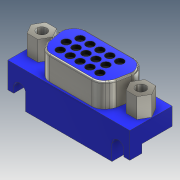
# Autodesk Inventor part: db15-connector-pcb
Saved by Autodesk Inventor 2017 (Build 210142000, 142)
## iProperties
Created: 2018-07-16
Part Number: db15-connector-pcb
Material: Generic
Document SubType Name: Modeling
Designer: Luiz Gustavo
Density: 1 g/cm^3
Appearance: Default
Author: Luiz Gustavo
Autodesk Inventor part; units mm, degrees
ref_plane "YZ Plane" through (0, 0, 0) normal (1, 0, 0) x (0, 1, 0)
ref_plane "XZ Plane" through (0, 0, 0) normal (0, 1, 0) x (-1, 0, 0)
ref_plane "XY Plane" through (0, 0, 0) normal (0, 0, 1) x (1, 0, 0)
sketch "Sketch1" plane through (0, 0, 0) normal (0, 0, 1) x (1, 0, 0)
  line L0 (-15.4, 5.35) -> (15.4, 5.35)
  line L1 (15.4, 5.35) -> (15.4, -5.35)
  line L2 (15.4, -5.35) -> (-15.4, -5.35)
  line L3 (-15.4, -5.35) -> (-15.4, 5.35)
  line L4 (-15.4, 5.35) -> (15.4, -5.35) construction
  line L5 (15.4, 5.35) -> (-15.4, -5.35) construction
  line L6 (-15.4, 0.35) -> (15.4, 0.35) construction
  circle A0 centre (-12.5, 0.35) radius 1.25
  circle A1 centre (12.5, 0.35) radius 1.25
  line L7 (0, 5.35) -> (0, -5.35) construction
  circle A2 centre (-12.5, 0.35) radius 2.7424 construction
  line L8 (-13.8712, -2.025) -> (-11.1288, 2.725) construction
  line L9 (-13.8712, 2.725) -> (-11.1288, -2.025) construction
  line L10 (-9.7576, 0.35) -> (-15.2424, 0.35) construction
  line L11 (-11.1288, 2.725) -> (-13.8712, 2.725)
  line L12 (-13.8712, 2.725) -> (-15.2424, 0.35)
  line L13 (-15.2424, 0.35) -> (-13.8712, -2.025)
  line L14 (-13.8712, -2.025) -> (-11.1288, -2.025)
  line L15 (-11.1288, -2.025) -> (-9.7576, 0.35)
  line L16 (-9.7576, 0.35) -> (-11.1288, 2.725)
  line L17 (11.1288, 2.725) -> (13.8712, 2.725)
  line L18 (13.8712, 2.725) -> (15.2424, 0.35)
  line L19 (15.2424, 0.35) -> (13.8712, -2.025)
  line L20 (13.8712, -2.025) -> (11.1288, -2.025)
  line L21 (11.1288, -2.025) -> (9.7576, 0.35)
  line L22 (9.7576, 0.35) -> (11.1288, 2.725)
  line L23 (-7.5, 5.15) -> (7.5, 5.15)
  line L24 (7.5, 5.15) -> (9.5, 2.55)
  line L25 (9.5, 2.55) -> (8.5, -2.65)
  line L26 (8.5, -2.65) -> (6.75, -4.85)
  line L27 (6.75, -4.85) -> (-6.75, -4.85)
  line L28 (-6.75, -4.85) -> (-8.5, -2.65)
  line L29 (-8.5, -2.65) -> (-9.5, 2.55)
  line L30 (-9.5, 2.55) -> (-7.5, 5.15)
  point P0 (0, 0)
  dimension "d0" = 30.8
  dimension "d1" = 10.7
  dimension "d2" = 2.5
  dimension "d4" = 60
  dimension "d5" = 60
  dimension "d6" = 4.75
  dimension "d7" = 5
  dimension "d8" = 25
  dimension "d9" = 15
  dimension "d10" = 19
  dimension "d11" = 13.5
  dimension "d12" = 17
  dimension "d13" = 10
  dimension "d14" = 7.4
  dimension "d15" = 2.2
  dimension "d16" = 0.2
  constraints: 62 end point, 10 symmetric about line, 7 midpoint, 6 parallel, 6 point on circle, 4 horizontal, 4 point on line, 3 centre point, 1 perpendicular, 1 other
  measures "d0" distance of L1.end L2.end
  measures "d1" distance of L0.end L1.end
  measures "d2" diameter of A0
  measures "d4" angle of L9 L8
  measures "d5" angle of L9 L10
  measures "d6" distance between parallel lines of L14 L11
  measures "d7" distance between parallel lines of L6 L0
  measures "d8" distance of A1.centre A0.centre
  measures "d9" distance of L23.start L23.end
  measures "d10" distance of L24.end L29.end
  measures "d11" distance of L26.end L27.end
  measures "d12" distance of L25.end L28.end
  measures "d13" distance between parallel lines of L27 L23
  measures "d14" distance from line of L29.end L27
  measures "d15" vertical distance of L26.end L25.end
  measures "d16" distance between parallel lines of L23 L0
extrude "Extrusion1" add sketch "Sketch1" along normal blind 5 contours L16 L15 L14 L13 L12 L11 | L17 L18 L19 L20 L21 L22
extrude "Extrusion2" add sketch "Sketch1" along normal blind 6 contours L23 L24 L25 L26 L27 L28 L29 L30
extrude "Extrusion3" add sketch "Sketch1" against normal blind 9 contours L0 L1 L2 L3 | A0 | A1 | L16 L15 L14 L13 L12 L11 | L17 L18 L19 L20 L21 L22 | L23 L24 L25 L26 L27 L28 L29 L30
sketch "Sketch2" plane through (-15.4, 5.35, 0) normal (0, 1, 0) x (1, 0, 0)
  line L0 (0, 0) -> (30.8, 0) projected
  line L1 (30.8, 0) -> (30.8, 9) projected
  line L2 (0, 9) -> (30.8, 9) projected
  line L3 (0, 0) -> (0, 9) projected
  line L4 (15.4, 0) -> (15.4, 9) construction
  line L5 (0, 0) -> (0, 9) projected
  line L6 (0, 9) -> (6.9, 9)
  line L7 (6.9, 9) -> (6.9, 4.4)
  line L8 (6.9, 4.4) -> (0, 4.4)
  line L9 (0, 4.4) -> (0, 9)
  line L10 (30.8, 9) -> (0, 9) projected
  line L11 (30.8, 9) -> (23.9, 9)
  line L12 (23.9, 9) -> (23.9, 4.4)
  line L13 (23.9, 4.4) -> (30.8, 4.4)
  line L14 (30.8, 4.4) -> (30.8, 9)
  line L15 (6.9, 4.4) -> (23.9, 4.4) construction
  dimension "d23" = 17
  dimension "d24" = 4.4
  constraints: 20 end point, 4 parallel, 3 perpendicular, 2 horizontal, 1 midpoint, 1 point on line, 1 other
  measures "d23" distance between parallel lines of L12 L7
  measures "d24" distance between parallel lines of L0 L15
extrude "Extrusion4" cut sketch "Sketch2" against normal blind 7.7 contours L3 L2 L7 L8 | L13 L12 L2 L1
sketch "Sketch3" plane through (0, 0, 6) normal (0, 0, 1) x (1, 0, 0)
  line L0 (-5, 2.5) -> (3.2977, 2.5) construction
  circle A0 centre (-5, 2.5) radius 1
  circle A1 centre (-2.5, 2.5) radius 1
  circle A2 centre (0, 2.5) radius 1
  circle A3 centre (2.5, 2.5) radius 1
  circle A4 centre (5, 2.5) radius 1
  line L1 (-6, 0) -> (3.7977, 0) construction
  circle A5 centre (-6, 0) radius 1
  circle A6 centre (-3.5, 0) radius 1
  circle A7 centre (-1, 0) radius 1
  circle A8 centre (1.5, 0) radius 1
  circle A9 centre (4, 0) radius 1
  line L2 (-5, -2.5) -> (3.1289, -2.5) construction
  circle A10 centre (-5, -2.5) radius 1
  circle A11 centre (-2.5, -2.5) radius 1
  circle A12 centre (0, -2.5) radius 1
  circle A13 centre (2.5, -2.5) radius 1
  circle A14 centre (5, -2.5) radius 1
  line L3 (0, 2.5) -> (0, -2.5) construction
  point P0 (0, 0)
  point P1 (0, 0)
  dimension "d27" = 2
  dimension "d30" = 2.5
  dimension "d39" = 2
  dimension "d40" = 2.5
  dimension "d50" = 2
  dimension "d51" = 2.5
  dimension "d53" = 2.5
  dimension "d54" = 2.5
  constraints: 15 centre point, 8 end point, 6 horizontal, 4 coincident, 1 midpoint, 1 tangent, 1 vertical, 24 other
  measures "d27" diameter of A0
  measures "d30" distance of A0.centre A1.centre
  measures "d39" diameter of A5
  measures "d40" distance of A5.centre A6.centre
  measures "d50" diameter of A10
  measures "d51" distance of A10.centre A11.centre
  measures "d53" vertical distance of A9.centre A4.centre
  measures "d54" vertical distance of A14.centre A9.centre
extrude "Extrusion5" cut sketch "Sketch3" against normal blind 1
fillet "Fillet1" radius 3 8 edges at (-7.5, 5.15, 3) (-9.5, 2.55, 3) (-8.5, -2.65, 3) (-6.75, -4.85, 3) (6.75, -4.85, 3) (8.5, -2.65, 3) (9.5, 2.55, 3) (7.5, 5.15, 3)
sketch "Sketch4" plane through (0, 0, 0) normal (0, 1, 0) x (-1, 0, 0)
  line L0 (-15.4, -9) -> (15.4, -9) projected
  line L1 (15.4, -4.4) -> (15.4, -9) projected
  line L2 (-15.4, -9) -> (-15.4, -4.4) projected
  line L3 (15.4, -6.5) -> (13.9, -6.5)
  line L4 (13.9, -6.5) -> (13.9, -5)
  line L5 (10.9, -5) -> (10.9, -9)
  line L6 (10.9, -9) -> (15.4, -9)
  line L7 (15.4, -9) -> (15.4, -6.5)
  arc A0 (13.9, -5) -> (10.9, -5) centre (12.4, -5) ccw
  line L8 (8.5, -9) -> (-8.5, -9) projected
  line L9 (0, -9) -> (0, -5) construction
  arc A1 (10.9, -5) -> (13.9, -5) centre (12.4, -5) ccw construction
  line L10 (-15.4, -4.4) -> (-15.4, -9)
  line L11 (-15.4, -6.5) -> (-13.9, -6.5)
  line L12 (-13.9, -6.5) -> (-13.9, -5)
  line L13 (-10.9, -5) -> (-10.9, -9)
  line L14 (-10.9, -9) -> (-15.4, -9)
  line L15 (-15.4, -9) -> (-15.4, -6.5)
  arc A2 (-10.9, -5) -> (-13.9, -5) centre (-12.4, -5) ccw
  arc A3 (-13.9, -5) -> (-10.9, -5) centre (-12.4, -5) ccw construction
  point P0 (0, 0)
  dimension "d58" = 3
  dimension "d59" = 4
  dimension "d60" = 3
  dimension "d61" = 2.5
  constraints: 24 end point, 8 point on circle, 6 symmetric about line, 4 centre point, 3 perpendicular, 3 point on line, 2 tangent, 1 collinear, 1 horizontal, 1 midpoint, 1 vertical, 2 other
  measures "d58" diameter of A0
  measures "d59" distance from line of L0 A0.centre
  measures "d60" horizontal distance of L3.start A0.centre
  measures "d61" distance between parallel lines of L3 L0
extrude "Extrusion6" cut sketch "Sketch4" against normal through all
fillet "Fillet2" radius 0.4 16 edges at (-7.3481, 4.8414, 6) (-8.5388, 3.7996, 6) (-9.2181, 2.4831, 6) (-8.9421, -0.3508, 6) (-8.4189, -2.6127, 6) (-7.8459, -3.4723, 6) (-6.6063, -4.5521, 6) (0, -4.85, 6) (6.6063, -4.5521, 6) (7.8459, -3.4723, 6) (8.4189, -2.6127, 6) (8.9421, -0.3508, 6) (9.2181, 2.4831, 6) (8.5388, 3.7996, 6) (7.3481, 4.8414, 6) (0, 5.15, 6)
equation "\"d5\" = d4"
equation "\"d54\" = d53"
body "Solid1"
